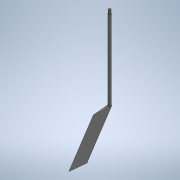
# Autodesk Inventor part: rudder_pair_queens
Saved by Autodesk Inventor 2020 (Build 240168000, 168)
## iProperties
Created: 2019-09-18
Part Number: rudder_pair_queens
Material: Generic
Document SubType Name: Modeling
Designer: suchanek
Density: 1 g/cm^3
Appearance: Default
Author: suchanek
Autodesk Inventor part; units mm, degrees
ref_plane "YZ Plane" through (0, 0, 0) normal (1, 0, 0) x (0, 1, 0)
ref_plane "XZ Plane" through (0, 0, 0) normal (0, 1, 0) x (-1, 0, 0)
ref_plane "XY Plane" through (0, 0, 0) normal (0, 0, 1) x (1, 0, 0)
sketch "Sketch1" plane through (0, 0, 0) normal (0, 1, 0) x (-1, 0, 0)
  arc A0 (-3.9799, 0.4) -> (3.9799, 0.4) centre (0, 0) ccw
  line L0 (-3.9799, 0.4) -> (0, 40)
  line L1 (0, 40) -> (3.9799, 0.4)
  dimension "d0" = 4
  dimension "d1" = 40
  constraints: 4 end point, 2 point on circle, 2 tangent, 1 centre point, 1 coincident, 1 vertical alignment
  measures "d0" radius of A0
  measures "d1" distance of L0.end point (0, 0)
sketch "Sketch2" plane through (0, 0, 0) normal (1, 0, 0) x (0, 1, 0)
  line L0 (0, 0) -> (-90, 60)
  dimension "d2" = 90
  dimension "d3" = 60
  constraints: 2 end point
  measures "d2" horizontal distance of L0.end L0.start
  measures "d3" vertical distance of L0.start L0.end
sweep "Sweep1" add profiles "Sketch1" path "Sketch2"
sketch "Sketch3" plane through (0, 0, 0) normal (0, 1, 0) x (1, 0, 0)
  circle A0 centre (0, 0) radius 3.5
  dimension "d6" = 7
  constraints: 1 centre point, 1 coincident
  measures "d6" diameter of A0
extrude "Extrusion1" add sketch "Sketch3" along normal blind 204
sketch "Sketch4" plane through (0, 204, 0) normal (0, 1, 0) x (1, 0, 0)
  circle A0 centre (0, 0) radius 3
  circle A1 centre (0, 0) radius 5
  line L0 (-0.5, -5) -> (0.5, -5)
  line L1 (0.5, -5) -> (0.5, 5)
  line L2 (0.5, 5) -> (-0.5, 5)
  line L3 (-0.5, 5) -> (-0.5, -5)
  line L4 (-0.5, -5) -> (0.5, 5) construction
  line L5 (0.5, -5) -> (-0.5, 5) construction
  point P0 (-0.5, -2.958)
  point P1 (-0.5, 2.958)
  point P2 (0.5, 2.958)
  point P3 (0.5, -2.958)
  dimension "d9" = 6
  dimension "d10" = 10
  dimension "d11" = 1
  dimension "d12" = 10
  constraints: 12 end point, 2 centre point, 2 coincident, 2 midpoint, 2 parallel, 1 horizontal, 1 perpendicular
  measures "d9" diameter of A0
  measures "d10" diameter of A1
  measures "d11" distance of L2.end L1.end
  measures "d12" distance of L1.end L0.end
extrude "Extrusion2" cut sketch "Sketch4" against normal blind 10 contours A0 L1 A1 | L1 A0 L3 | A0 L3 A1 L1 | L1 A1 L3 A0 | A0 L3 A1
thread "Thread1"
body "Solid1"
